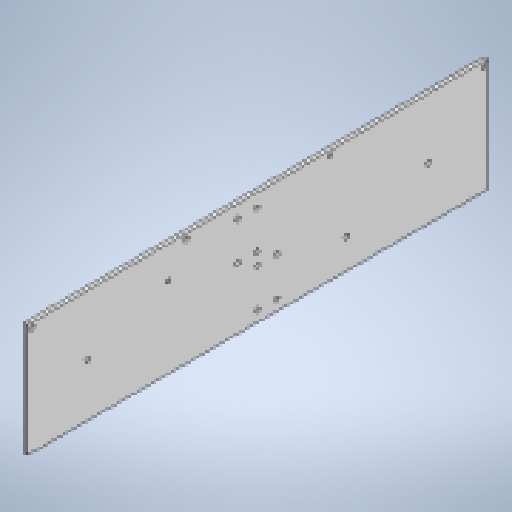
# Autodesk Inventor part: InsideChassiPlate4.0
Saved by Autodesk Inventor 2023 (Build 270158000, 158)
## iProperties
Created: 2022-09-29
Part Number: InsideChassiPlate4.0
Material: Generic
Document SubType Name: Modeling
Designer: deli
Density: 1 g/cm^3
Appearance: Default
Author: deli
Autodesk Inventor part; units mm, degrees
ref_plane "YZ Plane" through (0, 0, 0) normal (1, 0, 0) x (0, 1, 0)
ref_plane "XZ Plane" through (0, 0, 0) normal (0, 1, 0) x (-1, 0, 0)
ref_plane "XY Plane" through (0, 0, 0) normal (0, 0, 1) x (1, 0, 0)
sketch "Sketch1" plane through (0, 0, 0) normal (1, 0, 0) x (0, 1, 0)
  line L0 (9.3448, 271.1671) -> (-84.6552, 271.1671)
  line L1 (-84.6552, 271.1671) -> (-84.6552, -112.8329)
  line L2 (-84.6552, -112.8329) -> (9.3448, -112.8329)
  line L3 (9.3448, -112.8329) -> (9.3448, 271.1671)
  circle A0 centre (-40.6552, 221.1671) radius 2
  circle A1 centre (-40.6552, -62.8329) radius 2
  circle A2 centre (-40.6552, 221.1671) radius 48 construction
  circle A3 centre (-40.6552, -62.8329) radius 48 construction
  circle A4 centre (5.3448, 267.1671) radius 2
  circle A5 centre (-1.7052, 96.0582) radius 1.9844
  circle A6 centre (-1.7052, 80.0582) radius 1.9844
  circle A7 centre (-33.7052, 80.0582) radius 1.9844
  circle A8 centre (-33.7052, 96.0582) radius 1.9844
  line L4 (-1.7052, 96.0582) -> (-1.7052, 80.0582) construction
  line L5 (-1.7052, 80.0582) -> (-33.7052, 80.0582) construction
  line L6 (-33.7052, 80.0582) -> (-33.7052, 96.0582) construction
  line L7 (-33.7052, 96.0582) -> (-1.7052, 96.0582) construction
  line L8 (1.3448, 102.7892) -> (-36.7552, 102.7892) construction
  line L9 (-36.7552, 102.7892) -> (-36.7552, 63.0382) construction
  line L10 (-36.7552, 63.0382) -> (1.3448, 63.0382) construction
  line L11 (1.3448, 63.0382) -> (1.3448, 102.7892) construction
  line L12 (-0.4332, 102.7892) -> (-34.9772, 102.7892) construction
  line L13 (-34.9772, 102.7892) -> (-34.9772, 112.0612) construction
  line L14 (-34.9772, 112.0612) -> (-0.4332, 112.0612) construction
  line L15 (-0.4332, 112.0612) -> (-0.4332, 102.7892) construction
  line L16 (-12.3712, 112.0612) -> (-23.0392, 112.0612) construction
  line L17 (-23.0392, 112.0612) -> (-23.0392, 120.0612) construction
  line L18 (-23.0392, 120.0612) -> (-12.3712, 120.0612) construction
  line L19 (-12.3712, 120.0612) -> (-12.3712, 112.0612) construction
  line L20 (-13.7052, 120.0612) -> (-21.7052, 120.0612) construction
  line L21 (-21.7052, 120.0612) -> (-21.7052, 123.0612) construction
  line L22 (-21.7052, 123.0612) -> (-13.7052, 123.0612) construction
  line L23 (-13.7052, 123.0612) -> (-13.7052, 120.0612) construction
  line L24 (1.2948, 63.0382) -> (-36.7052, 63.0382) construction
  line L25 (-36.7052, 63.0382) -> (-36.7052, -11.9618) construction
  line L26 (-36.7052, -11.9618) -> (1.2948, -11.9618) construction
  line L27 (1.2948, -11.9618) -> (1.2948, 63.0382) construction
  line L28 (-10.4552, 137.5612) -> (-24.9552, 137.5612) construction
  line L29 (-24.9552, 137.5612) -> (-29.7052, 132.5612) construction
  line L30 (-5.7052, 132.5612) -> (-10.4552, 137.5612) construction
  line L31 (-8.3552, 123.0612) -> (-27.0552, 123.0612) construction
  line L32 (-27.0552, 123.0612) -> (-27.0552, 132.5612) construction
  line L33 (-27.0552, 132.5612) -> (-8.3552, 132.5612) construction
  line L34 (-8.3552, 132.5612) -> (-8.3552, 123.0612) construction
  line L35 (-29.7052, 132.5612) -> (-5.7052, 132.5612) construction
  circle A9 centre (-17.7052, 154.1612) radius 21 construction
  circle A10 centre (-17.7052, 154.1612) radius 2
  circle A11 centre (-17.7052, 154.1612) radius 23.8732 construction
  circle A12 centre (-40.6552, 221.1671) radius 11.9366 construction
  line L36 (-30.176, 226.8827) -> (3.2532, 165.5925) construction
  line L37 (-41.2711, 150.3426) -> (-52.4382, 219.2577) construction
  circle A13 centre (-73.6052, 64.0391) radius 1.9844
  circle A14 centre (-73.6052, 80.0391) radius 1.9844
  circle A15 centre (-41.6052, 80.0391) radius 1.9844
  circle A16 centre (-41.6052, 64.0391) radius 1.9844
  line L38 (-73.6052, 64.0391) -> (-73.6052, 80.0391) construction
  line L39 (-73.6052, 80.0391) -> (-41.6052, 80.0391) construction
  line L40 (-41.6052, 80.0391) -> (-41.6052, 64.0391) construction
  line L41 (-41.6052, 64.0391) -> (-73.6052, 64.0391) construction
  line L42 (-76.6552, 57.3081) -> (-38.5552, 57.3081) construction
  line L43 (-38.5552, 57.3081) -> (-38.5552, 97.0591) construction
  line L44 (-38.5552, 97.0591) -> (-76.6552, 97.0591) construction
  line L45 (-76.6552, 97.0591) -> (-76.6552, 57.3081) construction
  line L46 (-74.8772, 57.3081) -> (-40.3332, 57.3081) construction
  line L47 (-40.3332, 57.3081) -> (-40.3332, 48.0361) construction
  line L48 (-40.3332, 48.0361) -> (-74.8772, 48.0361) construction
  line L49 (-74.8772, 48.0361) -> (-74.8772, 57.3081) construction
  line L50 (-62.9392, 48.0361) -> (-52.2712, 48.0361) construction
  line L51 (-52.2712, 48.0361) -> (-52.2712, 40.0361) construction
  line L52 (-52.2712, 40.0361) -> (-62.9392, 40.0361) construction
  line L53 (-62.9392, 40.0361) -> (-62.9392, 48.0361) construction
  line L54 (-61.6052, 40.0361) -> (-53.6052, 40.0361) construction
  line L55 (-53.6052, 40.0361) -> (-53.6052, 37.0361) construction
  line L56 (-53.6052, 37.0361) -> (-61.6052, 37.0361) construction
  line L57 (-61.6052, 37.0361) -> (-61.6052, 40.0361) construction
  line L58 (-76.6052, 97.0591) -> (-38.6052, 97.0591) construction
  line L59 (-38.6052, 97.0591) -> (-38.6052, 172.0591) construction
  line L60 (-38.6052, 172.0591) -> (-76.6052, 172.0591) construction
  line L61 (-76.6052, 172.0591) -> (-76.6052, 97.0591) construction
  line L62 (-64.8552, 22.5361) -> (-50.3552, 22.5361) construction
  line L63 (-50.3552, 22.5361) -> (-45.6052, 27.5361) construction
  line L64 (-69.6052, 27.5361) -> (-64.8552, 22.5361) construction
  line L65 (-63.8282, 37.0361) -> (-51.3822, 37.0361) construction
  line L66 (-51.3822, 37.0361) -> (-51.3822, 27.5361) construction
  line L67 (-51.3822, 27.5361) -> (-63.8282, 27.5361) construction
  line L68 (-63.8282, 27.5361) -> (-63.8282, 37.0361) construction
  line L69 (-45.6052, 27.5361) -> (-69.6052, 27.5361) construction
  circle A17 centre (-57.6052, 5.9361) radius 21 construction
  circle A18 centre (-57.6052, 5.9361) radius 2
  circle A19 centre (-57.6052, 5.9361) radius 23.8732 construction
  circle A20 centre (-40.6552, -62.8329) radius 11.9366 construction
  line L70 (-33.7944, 7.6611) -> (-28.7498, -61.9704) construction
  line L71 (-51.5978, -67.6019) -> (-79.4904, -3.6019) construction
  circle A21 centre (5.3448, -108.8329) radius 2
  circle A22 centre (5.3448, 131.1671) radius 2
  circle A23 centre (5.3448, 27.1671) radius 2
  point P0 (0, 0)
  point P1 (-62.9613, -17.3286)
  point P2 (-51.822, 29.0982)
  dimension "d0" = 384
  dimension "d1" = 4
  dimension "d2" = 4
  dimension "d3" = 50
  dimension "d4" = 50
  dimension "d5" = 44
  dimension "d6" = 96
  dimension "d7" = 96
  dimension "d8" = 50
  dimension "d9" = 50
  dimension "d10" = 4
  dimension "d11" = 4
  dimension "d12" = 4
  dimension "d13" = 3.9688
  dimension "d14" = 3.9688
  dimension "d15" = 3.9688
  dimension "d16" = 3.9688
  dimension "d17" = 16
  dimension "d18" = 32
  dimension "d19" = 38.1
  dimension "d20" = 3.05
  dimension "d21" = 39.751
  dimension "d22" = 6.731
  dimension "d23" = 34.544
  dimension "d24" = 1.778
  dimension "d25" = 9.272
  dimension "d26" = 10.668
  dimension "d27" = 8
  dimension "d28" = 13.716
  dimension "d29" = 8
  dimension "d30" = 3
  dimension "d32" = 15.05
  dimension "d33" = 38
  dimension "d34" = 0.05
  dimension "d35" = 75
  dimension "d38" = 18.7
  dimension "d39" = 9.7
  dimension "d42" = 14.5
  dimension "d45" = 24
  dimension "d46" = 7.05
  dimension "d47" = 14.5
  dimension "d48" = 42
  dimension "d49" = 19.05
  dimension "d50" = 16.6
  dimension "d51" = 4
  dimension "d52" = 47.7465
  dimension "d53" = 23.8732
  dimension "d54" = 160.595
  dimension "d55" = 160.595
  dimension "d56" = 69.814
  dimension "d57" = 3.9688
  dimension "d58" = 3.9688
  dimension "d59" = 3.9688
  dimension "d60" = 3.9688
  dimension "d61" = 16
  dimension "d62" = 32
  dimension "d63" = 38.1
  dimension "d64" = 3.05
  dimension "d65" = 39.751
  dimension "d66" = 6.731
  dimension "d67" = 34.544
  dimension "d68" = 1.778
  dimension "d69" = 9.272
  dimension "d70" = 10.668
  constraints: 144 end point, 28 parallel, 24 centre point, 19 perpendicular, 12 point on line, 10 horizontal, 10 point on circle, 8 coincident, 8 tangent, 2 equal length, 2 vertical, 1 collinear
  measures "d0" distance of L2.end L0.start
  measures "d1" diameter of A0
  measures "d2" diameter of A1
  measures "d3" distance from line of L3 A0.centre
  measures "d4" distance from line of L3 A1.centre
  measures "d5" distance from line of A0.centre L1
  measures "d6" diameter of A2
  measures "d7" diameter of A3
  measures "d8" distance from line of L0 A2.centre
  measures "d9" distance from line of L2 A1.centre
  measures "d10" diameter of A4
  measures "d11" distance from line of A4.centre L3
  measures "d12" distance from line of L0 A4.centre
  measures "d13" diameter of A5
  measures "d14" diameter of A6
  measures "d15" diameter of A8
  measures "d16" diameter of A7
  measures "d17" distance of L4.start L4.end
  measures "d18" distance of L6.end L4.start
  measures "d19" distance of L10.end L9.end
  measures "d20" distance from line of L4.start L11
  measures "d21" distance of L10.end L8.start
  measures "d22" distance from line of L4.start L8
  measures "d23" distance of L13.end L14.end
  measures "d24" distance between parallel lines of L11 L15
  measures "d25" distance of L14.end L12.start
  measures "d26" distance of L17.end L18.end
  measures "d27" distance of L16.end L17.end
  measures "d28" distance between parallel lines of L11 L19
  measures "d29" distance of L21.end L22.end
  measures "d30" distance of L20.end L21.end
  measures "d32" distance between parallel lines of L11 L23
  measures "d33" distance of L26.end L25.end
  measures "d34" distance between parallel lines of L11 L27
  measures "d35" distance of L26.end L24.start
  measures "d38" distance of L32.end L33.end
  measures "d39" distance between parallel lines of L11 L34
  measures "d42" distance between parallel lines of L31 L28
  measures "d45" distance of L29.end L30.start
  measures "d46" distance from line of L11 L30.start
  measures "d47" distance of L28.start L28.end
  measures "d48" diameter of A9
  measures "d49" distance from line of L11 A9.centre
  measures "d50" distance from line of L28 A9.centre
  measures "d51" diameter of A10
  measures "d52" diameter of A11
  measures "d53" diameter of A12
  measures "d56" distance of L36.start L36.end
  measures "d57" diameter of A13
  measures "d58" diameter of A14
  measures "d59" diameter of A16
  measures "d60" diameter of A15
  measures "d61" distance of L38.start L38.end
  measures "d62" distance of L40.end L38.start
  measures "d63" distance of L44.end L44.start
  measures "d64" distance from line of L38.start L45
  measures "d65" distance of L44.end L42.start
  measures "d66" distance from line of L38.start L42
  measures "d67" distance of L47.end L48.end
  measures "d68" distance between parallel lines of L45 L49
  measures "d69" distance of L48.end L46.start
  measures "d70" distance of L51.end L53.start
extrude "Extrusion1" add sketch "Sketch1" along normal blind 3.175
equation "\"d4\" = d3"
equation "\"d9\" = d8"
equation "\"d12\" = d11"
equation "\"d14\" = d13"
equation "\"d15\" = d13"
equation "\"d16\" = d13"
equation "\"d20\" = -0.5 * d18 + 0.5 * d19"
equation "\"d24\" = -0.5 * d23 + 0.5 * d19"
equation "\"d28\" = -0.5 * d26 + 0.5 * d19"
equation "\"d32\" = -0.5 * d29 + 0.5 * d19"
equation "\"d34\" = -0.5 * d33 + 0.5 * d19"
equation "\"d39\" = -0.5 * d38 + 0.5 * d19"
equation "\"d46\" = -0.5 * d45 + 0.5 * d19"
equation "\"d49\" = 0.5 * d19"
body "Solid1"
